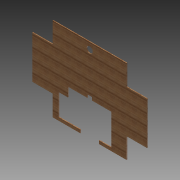
# Autodesk Inventor part: belly pan
Saved by Autodesk Inventor 2012 (Build 160160000, 160)
## iProperties
Created: 2013-10-07
Part Number: belly pan
Material: Default
Document SubType Name: Modeling
Designer: Bryce
Density: 1 g/cm^3
Author: Bryce
Autodesk Inventor part; units mm, degrees
ref_plane "YZ Plane" through (0, 0, 0) normal (1, 0, 0) x (0, 1, 0)
ref_plane "XZ Plane" through (0, 0, 0) normal (0, 1, 0) x (-1, 0, 0)
ref_plane "XY Plane" through (0, 0, 0) normal (0, 0, 1) x (1, 0, 0)
sketch "Sketch1" plane through (0, 0, 0) normal (0, 0, 1) x (1, 0, 0)
  line L0 (0, 0) -> (168.275, 0) construction
  line L1 (939.8, 0) -> (939.8, 168.275) construction
  line L2 (939.8, 685.8) -> (771.525, 685.8) construction
  line L3 (0, 685.8) -> (0, 517.525) construction
  line L4 (168.275, 517.525) -> (771.525, 517.525) construction
  line L5 (771.525, 517.525) -> (771.525, 168.275) construction
  line L6 (771.525, 168.275) -> (168.275, 168.275) construction
  line L7 (168.275, 168.275) -> (168.275, 517.525) construction
  line L8 (168.275, 517.525) -> (168.275, 685.8)
  line L9 (168.275, 517.525) -> (0, 517.525)
  line L10 (771.525, 517.525) -> (771.525, 685.8)
  line L11 (771.525, 517.525) -> (939.8, 517.525)
  line L12 (771.525, 168.275) -> (939.8, 168.275)
  line L13 (771.525, 168.275) -> (771.525, 0)
  line L14 (168.275, 168.275) -> (168.275, 0)
  line L15 (168.275, 168.275) -> (0, 168.275)
  line L16 (771.525, 685.8) -> (168.275, 685.8)
  line L17 (168.275, 685.8) -> (0, 685.8) construction
  line L18 (939.8, 517.525) -> (939.8, 685.8) construction
  line L19 (168.275, 0) -> (393.7, 0)
  line L20 (771.525, 0) -> (939.8, 0) construction
  line L21 (0, 168.275) -> (0, 0) construction
  line L22 (0, 517.525) -> (0, 168.275)
  line L23 (939.8, 168.275) -> (939.8, 517.525)
  line L24 (393.7, 0) -> (393.7, 25.4)
  line L25 (546.1, 0) -> (546.1, 25.4)
  line L26 (393.7, 25.4) -> (215.9, 25.4)
  line L27 (292.1, 203.2) -> (292.1, 279.4)
  line L28 (647.7, 279.4) -> (647.7, 25.4)
  line L29 (647.7, 25.4) -> (546.1, 25.4)
  line L30 (546.1, 0) -> (771.525, 0)
  line L31 (393.7, 0) -> (546.1, 0) construction
  line L32 (450.85, 279.4) -> (450.85, 304.8)
  line L33 (450.85, 304.8) -> (488.95, 304.8)
  line L34 (488.95, 304.8) -> (488.95, 279.4)
  line L35 (292.1, 279.4) -> (450.85, 279.4)
  line L36 (488.95, 279.4) -> (647.7, 279.4)
  circle A0 centre (469.9, 628.65) radius 25.4
  line L37 (292.1, 203.2) -> (215.9, 203.2)
  line L38 (215.9, 203.2) -> (215.9, 25.4)
  point P0 (469.9, 685.8)
  dimension "d0" = 939.8
  dimension "d1" = 685.8
  dimension "d2" = 603.25
  dimension "d3" = 349.25
  dimension "d4" = 168.275
  dimension "d5" = 168.275
  dimension "d6" = 168.275
  dimension "d8" = 168.275
  dimension "d11" = 152.4
  dimension "d12" = 225.425
  dimension "d13" = 225.425
  dimension "d14" = 25.4
  dimension "d15" = 355.6
  dimension "d17" = 25.4
  dimension "d18" = 38.1
  dimension "d19" = 50.8
  dimension "d20" = 57.15
  dimension "d21" = 254
  dimension "d22" = 123.825
  dimension "d23" = 123.825
  dimension "d24" = 76.2
  dimension "d25" = 177.8
  constraints: 78 end point, 41 perpendicular, 32 parallel, 7 horizontal, 2 equal length, 2 point on line, 1 centre point, 1 collinear, 1 horizontal alignment, 1 midpoint, 1 vertical alignment
  measures "d0" distance of L0.start L1.start
  measures "d1" distance of L3.start L0.start
  measures "d2" distance of L4.start L4.end
  measures "d3" distance of L6.end L4.start
  measures "d4" distance of L4.start L8.end
  measures "d5" distance of L4.end L11.end
  measures "d6" distance of L5.end L13.end
  measures "d8" distance of L6.end L15.end
  measures "d11" distance between parallel lines of L25 L24
  measures "d12" distance between parallel lines of L14 L24
  measures "d13" distance between parallel lines of L25 L13
  measures "d14" distance of L19.end L24.end
  measures "d15" distance of L27.end L28.start
  measures "d17" distance of L32.start L32.end
  measures "d18" distance of L32.end L33.end
  measures "d19" diameter of A0
  measures "d20" distance from line of L16 A0.centre
  measures "d21" distance between parallel lines of L35 L26
  measures "d22" distance between parallel lines of L13 L28
  measures "d23" distance between parallel lines of L14 L27
  measures "d24" distance of L27.start L37.end
  measures "d25" distance of L37.end L26.end
extrude "Extrusion1" add sketch "Sketch1" along normal blind 6.35
equation "\"d4\" = d6"
equation "\"d5\" = d8"
equation "\"d12\" = d13"
equation "\"d22\" = d23"
body "Solid1"
